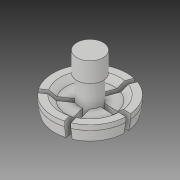
# Autodesk Inventor part: Top
Saved by Autodesk Inventor 2018 (Build 220112000, 112)
## iProperties
Created: 2017-12-12
Part Number: Top
Material: Generic
Document SubType Name: Modeling
Designer: Rus
Density: 1 g/cm^3
Appearance: Default
Author: Rus
Autodesk Inventor part; units mm, degrees
ref_plane "YZ Plane" through (0, 0, 0) normal (1, 0, 0) x (0, 1, 0)
ref_plane "XZ Plane" through (0, 0, 0) normal (0, 1, 0) x (-1, 0, 0)
ref_plane "XY Plane" through (0, 0, 0) normal (0, 0, 1) x (1, 0, 0)
sketch "Sketch1" plane through (0, 0, 0) normal (0, 0, 1) x (1, 0, 0)
  line L0 (0, 0) -> (0, 25.4)
  line L1 (0, 0) -> (0, -6.35)
  line L2 (0, 25.4) -> (0, 38.1)
  line L3 (8.4667, 25.4) -> (8.4667, 38.1)
  line L4 (8.4667, 38.1) -> (0, 38.1)
  line L5 (3.175, 17.0324) -> (0, 17.0324) construction
  line L6 (8.4667, 25.4) -> (6.8792, 25.4)
  line L7 (6.8792, 25.4) -> (0, 25.4) construction
  line L8 (0, 0) -> (3.175, 0) construction
  line L9 (3.175, 0) -> (17.91, 0) construction
  line L10 (22.6258, 3.4297) -> (23.8125, 10.16)
  line L11 (23.8125, 10.16) -> (23.8125, 13.335)
  line L12 (15.3458, 10.16) -> (6.8792, 10.16)
  line L13 (19.1558, 13.335) -> (23.8125, 13.335)
  line L14 (0, -6.35) -> (3.175, -4.2333)
  line L15 (3.175, -4.2333) -> (3.175, 0)
  line L16 (15.3458, 10.16) -> (19.1558, 13.335)
  line L17 (3.175, 0) -> (22.6258, 3.4297)
  line L18 (6.8792, 25.4) -> (6.8792, 10.16)
  dimension "d5" = 44.45
  dimension "d6" = 12.7
  dimension "d7" = 8.4667
  dimension "d12" = 2.1167
  dimension "d13" = 3.175
  dimension "d15" = 4.2333
  dimension "d18" = 3.175
  dimension "d20" = 3.175
  dimension "d21" = 3.81
  dimension "d23" = 10.16
  dimension "d24" = 10
  dimension "d26" = 23.8125
  dimension "d27" = 110
  dimension "d28" = 1.5875
  dimension "d29" = 8.4667
  constraints: 39 end point, 6 vertical, 4 horizontal, 3 perpendicular, 2 point on line
  measures "d5" distance of L2.end L1.end
  measures "d6" distance of L3.start L3.end
  measures "d7" distance between parallel lines of L2 L3
  measures "d12" vertical distance of L14.end L1.end
  measures "d13" horizontal distance of L1.end L14.end
  measures "d15" distance from line of L9 L14.end
  measures "d18" distance of L11.end L10.end
  measures "d20" distance between parallel lines of L12 L13
  measures "d21" horizontal distance of L13.start L12.start
  measures "d23" vertical distance of L12.start L9.end
  measures "d24" angle of L17 L9
  measures "d26" horizontal distance of L10.end L1.end
  measures "d27" angle of L17 L10
  measures "d28" distance of L3.start L6.end
  measures "d29" distance of L12.end L12.start
revolve "Revolution1" add sketch "Sketch1" angle 360 about axis through (0, 25.4, 0) along (0, -1, 0)
sketch "Sketch2" plane through (0, 13.335, 0) normal (0, 1, 0) x (1, 0, 0)
  line L0 (-0.6307, 7.5502) -> (5.1608, 23.4623)
  line L1 (5.1608, 23.4623) -> (8.1444, 22.3764)
  line L2 (8.1444, 22.3764) -> (2.3528, 6.4643)
  line L3 (2.3528, 6.4643) -> (-0.6307, 7.5502) construction
  circle A0 centre (0, 0) radius 6.8792 projected
  circle A1 centre (0, 0) radius 23.8125 projected
  line L4 (0, 0) -> (0, 6.8792) construction
  line L5 (-0.6307, 7.5502) -> (-0.8963, 6.8205)
  arc A2 (2.3528, 6.4643) -> (-0.8963, 6.8205) centre (0, 0) ccw
  point P0 (0, 0)
  dimension "d30" = 3.175
  dimension "d31" = 160
  constraints: 12 end point, 6 point on circle, 2 parallel, 1 centre point, 1 collinear, 1 perpendicular, 1 tangent, 1 vertical, 2 other
  measures "d30" distance between parallel lines of L0 L2
  measures "d31" angle of L2 L4
extrude "Extrusion1" cut sketch "Sketch2" against normal through all contours L0 A1 L2 A0 L5 | L0 L1 A1 picked at (1.917, 12.5231)
pattern_circular "Circular Pattern1" count 5 over 360 about axis through (0, 31.75, 0) along (0, -1, 0) of "Extrusion1"
body "Solid1"
